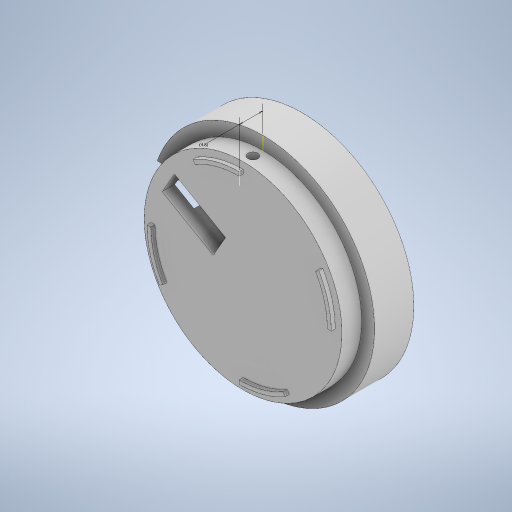
# Autodesk Inventor part: PiezoMount
Saved by Autodesk Inventor 2023 (Build 270158000, 158)
## iProperties
Created: 2023-02-27
Part Number: PiezoMount
Material: Generic
Document SubType Name: Modeling
Designer: maste
Density: 1 g/cm^3
Appearance: Default
Author: maste
Autodesk Inventor part; units mm, degrees
ref_plane "YZ Plane" through (0, 0, 0) normal (1, 0, 0) x (0, 1, 0)
ref_plane "XZ Plane" through (0, 0, 0) normal (0, 1, 0) x (-1, 0, 0)
ref_plane "XY Plane" through (0, 0, 0) normal (0, 0, 1) x (1, 0, 0)
sketch "Sketch1" plane through (0, 0, 0) normal (0, 0, 1) x (1, 0, 0)
  circle A0 centre (0, 0) radius 20.125
  dimension "d2" = 40.25
  constraints: 1 centre point, 1 coincident
  measures "d2" diameter of A0
extrude "piezo surface" add sketch "Sketch1" along normal blind 1
sketch "Sketch4" plane through (0, 0, 0) normal (0, 0, -1) x (-1, 0, 0)
  circle A0 centre (0, 0) radius 20.125 projected
extrude "Depth extension to surface" add sketch "Sketch4" along normal blind 6
sketch "Sketch2" plane through (0, 0, 1) normal (0, 0, 1) x (1, 0, 0)
  circle A0 centre (0, 0) radius 17.95
  circle A1 centre (0, 0) radius 18.75
  line L0 (0, 0) -> (18.75, 0)
  arc A2 (18.75, 0) -> (16.238, 9.375) centre (0, 0) ccw
  line L1 (0, 0) -> (16.238, 9.375) construction
  line L2 (0, 0) -> (18.75, 0) construction
  line L3 (16.238, 9.375) -> (15.5452, 8.975)
  line L4 (0, 0) -> (0, 18.75)
  line L5 (0, 0) -> (0, -18.75)
  line L6 (0, 0) -> (-18.75, 0)
  line L7 (0, 0) -> (-16.238, -9.375)
  line L8 (0, 0) -> (-9.375, 16.238)
  line L9 (0, 0) -> (9.375, -16.238)
  point P0 (17.95, 0)
  point P1 (8.975, -15.5452)
  point P2 (0, -17.95)
  point P3 (-15.5452, -8.975)
  point P4 (-17.95, 0)
  point P5 (-8.975, 15.5452)
  point P6 (0, 17.95)
  dimension "d3" = 35.9
  dimension "d4" = 37.5
  dimension "d5" = 30
  constraints: 20 end point, 4 point on line, 3 coincident, 2 perpendicular, 2 point on circle, 1 centre point, 1 horizontal, 1 vertical, 12 other
  measures "d5" angle of L2 L1
extrude "Diaphragm support" add sketch "Sketch2" along normal blind 0.8 contours A0 L3 A1 L0 | L9 A1 L5 A0 | A0 L8 A1 L4 | A0 L7 A1 L6
sketch "Sketch3" plane through (0, 0, 1) normal (0, 0, 1) x (1, 0, 0)
  line L0 (0, 0) -> (8.975, -15.5452)
  arc A0 (17.95, 0) -> (15.5452, 8.975) centre (0, 0) ccw projected
  line L1 (0, 0) -> (17.95, 0)
  arc A1 (0, -17.95) -> (8.975, -15.5452) centre (0, 0) ccw projected
  line L2 (8.975, -15.5452) -> (17.95, 0)
  line L3 (13.4625, -7.7726) -> (0, 0)
  line L4 (13.4625, -7.7726) -> (4.8022, -2.7726)
  line L5 (13.4625, -7.7726) -> (4.8022, -2.7726)
  line L6 (13.4625, -7.7726) -> (4.8022, -2.7726)
  line L7 (4.8022, -2.7726) -> (6.0522, -0.6075)
  line L8 (6.0522, -0.6075) -> (14.7125, -5.6075)
  line L9 (14.7125, -5.6075) -> (13.4625, -7.7726)
  line L10 (13.4625, -7.7726) -> (4.8022, -2.7726)
  line L11 (4.8022, -2.7726) -> (3.5522, -4.9376)
  line L12 (3.5522, -4.9376) -> (12.2125, -9.9376)
  line L13 (12.2125, -9.9376) -> (13.4625, -7.7726)
  line L14 (12.2125, -9.9376) -> (14.7125, -5.6075)
  line L15 (14.7125, -5.6075) -> (16.4446, -6.6075)
  line L16 (16.4446, -6.6075) -> (13.9446, -10.9376)
  line L17 (13.9446, -10.9376) -> (12.2125, -9.9376)
  line L18 (15.1946, -8.7726) -> (-15.1943, 8.7724)
  line L19 (-15.1943, 8.7724) -> (-4.802, 2.7724)
  line L20 (-4.802, 2.7724) -> (-3.552, 4.9375)
  line L21 (-3.552, 4.9375) -> (-13.9443, 10.9375)
  line L22 (-13.9443, 10.9375) -> (-15.1943, 8.7724)
  line L23 (-15.1943, 8.7724) -> (-4.802, 2.7724)
  line L24 (-4.802, 2.7724) -> (-6.052, 0.6074)
  line L25 (-6.052, 0.6074) -> (-16.4443, 6.6074)
  line L26 (-16.4443, 6.6074) -> (-15.1943, 8.7724)
  point P0 (14.7125, -5.6075)
  point P1 (12.2125, -9.9376)
  point P2 (12.2125, -9.9376)
  dimension "d37" = 10
  dimension "d38" = 2.5
  dimension "d39" = 2.5
  dimension "d40" = 2
  dimension "d49" = 10
  dimension "d50" = 35.09
  dimension "d51" = 12
  constraints: 54 end point, 10 parallel, 5 collinear, 5 perpendicular, 3 point on line, 2 midpoint
  measures "d37" distance of L3.start L4.end
  measures "d38" distance of L4.end L7.end
  measures "d39" distance of L11.end L4.end
  measures "d40" distance of L8.end L15.end
  measures "d49" distance between parallel lines of L11 L13
  measures "d50" distance of L18.start L18.end
  measures "d51" distance of L18.end L19.end
extrude "Microphone Wire Hole" cut sketch "Sketch3" against normal blind 14 contours L24 L25 L26 L18 | L18 L22 L21 L20
sketch "Sketch5" plane through (0, 0, -6) normal (0, 0, -1) x (-1, 0, 0)
  line L0 (12.5, -12.5) -> (-12.5, -12.5)
  line L1 (-12.5, -12.5) -> (-12.5, 12.5)
  line L2 (-12.5, 12.5) -> (12.5, 12.5)
  line L3 (12.5, 12.5) -> (12.5, -12.5)
  line L4 (12.5, -12.5) -> (-12.5, 12.5) construction
  line L5 (-12.5, -12.5) -> (12.5, 12.5) construction
  point P0 (0, 0)
  dimension "d18" = 25
  dimension "d19" = 25
  constraints: 12 end point, 2 midpoint, 2 parallel, 1 horizontal, 1 perpendicular
  measures "d18" distance of L0.start L0.end
  measures "d19" distance of L0.end L1.end
extrude "Circuit chamber" cut sketch "Sketch5" against normal blind 3
sketch "Sketch6" plane through (-12.5, -12.5, -6) normal (1, 0, 0) x (0, 0, -1)
  line L0 (0, 25) -> (0, 22.6036) projected
  line L1 (0, 25) -> (-3, 25) projected
  line L2 (-3, 25) -> (-3, 22.6036) projected
  line L3 (0, 0) -> (-3, 0) projected
  line L4 (-4.5, 5) -> (0, 5)
  line L5 (0, 5) -> (0, 20)
  line L6 (0, 20) -> (-4.5, 20)
  line L7 (-4.5, 20) -> (-4.5, 5)
  line L8 (-4.5, 5) -> (0, 20) construction
  line L9 (0, 5) -> (-4.5, 20) construction
  line L10 (0, 22.6036) -> (-3, 22.6036) projected
  line L11 (-3, 16.8301) -> (0, 16.8301) projected
  line L12 (-3, 16.8301) -> (-3, 0) projected
  line L13 (0, 16.8301) -> (0, 0) projected
  point P0 (-6, 12.5)
  point P1 (-2.25, 12.5)
  point P2 (-3, 20)
  point P3 (-3, 5)
  point P4 (0, 5)
  dimension "d22" = 15
  dimension "d45" = 5
  constraints: 12 end point, 2 midpoint, 2 parallel, 1 perpendicular
  measures "d22" distance of L5.end L4.end
  measures "d45" distance between parallel lines of L1 L6
extrude "port vent" cut sketch "Sketch6" against normal blind 30 contours L0 L10 L2 L1 | L4 L12 L11 L5 | L4 L7 L6 L5 L11 L12
sketch "Sketch7" plane through (0, 0, -6) normal (0, 0, -1) x (-1, 0, 0)
  line L0 (0, 0) -> (0, -17.5)
  line L1 (0, 0) -> (0, 17.5)
  dimension "d25" = 17.5
  dimension "d26" = 17.5
  constraints: 4 end point, 2 coincident, 2 vertical
  measures "d25" distance of L0.start L0.end
  measures "d26" distance of L0.start L1.end
hole "screw holes" at (0, 17.5, -6) at (0, -17.5, -6) direction (0, 0, 1) diameter 2.5 depth 4 tip angle 118
sketch "Sketch8" plane through (0, 0, -6) normal (0, 0, -1) x (-1, 0, 0)
  circle A0 centre (0, 0) radius 22.75
  line L0 (15.9289, 7.5) -> (18.6753, 7.5) projected
  line L1 (18.6753, 7.5) -> (21.4782, 7.5)
  arc A1 (18.6753, 7.5) -> (18.6753, -7.5) centre (0, 0) ccw projected
  line L2 (18.6753, -7.5) -> (21.4782, -7.5)
  point P0 (12.5, 7.5)
  dimension "d34" = 45.5
  constraints: 4 end point, 2 point on circle, 1 centre point, 1 coincident, 1 collinear, 1 parallel
  measures "d34" diameter of A0
extrude "Rim for flush with diaphragm lock" add sketch "Sketch8" against normal blind 3 contours L1 A1 L2 A0 picked at (-21.7141, -0.803)
sketch "Sketch9" plane through (0, 0, 0) normal (0, 1, 0) x (-1, 0, 0)
  line L0 (12.5, -3) -> (-12.5, -3) projected
  line L1 (0, -3) -> (0, -1)
  circle A0 centre (0, -1) radius 1
  point P0 (0, 0)
  dimension "d41" = 2
  dimension "d42" = 2
  constraints: 2 end point, 1 centre point, 1 coincident, 1 midpoint, 1 vertical
  measures "d41" distance of L1.start L1.end
  measures "d42" diameter of A0
extrude "Extrusion8" cut sketch "Sketch9" along normal mid plane 100
sketch "Sketch10" plane through (0, 0, -6) normal (0, 0, -1) x (-1, 0, 0)
  circle A0 centre (0, 17.5) radius 1.25 projected
  circle A1 centre (0, -17.5) radius 1.25 projected
  line L0 (15.9289, 7.5) -> (21.4782, 7.5) projected
  arc A2 (21.4782, 7.5) -> (21.4782, -7.5) centre (0, 0) ccw projected
  line L1 (21.4782, -7.5) -> (12.5, -7.5) projected
  line L2 (12.5, -7.5) -> (12.5, -12.5) projected
  line L3 (12.5, -12.5) -> (-12.5, -12.5) projected
  line L4 (-12.5, -12.5) -> (-12.5, 12.5) projected
  line L5 (-12.5, 12.5) -> (15.7723, 12.5) projected
  arc A3 (17.405, 10.1036) -> (15.7723, 12.5) centre (0, 0) ccw projected
  line L6 (17.405, 10.1036) -> (14.4257, 10.1036) projected
  line L7 (14.4257, 10.1036) -> (15.9289, 7.5) projected
extrude "Extrusion9" add sketch "Sketch10" along normal blind 5
sketch "Sketch11" plane through (0, 0, 0) normal (1, 0, 0) x (0, 1, 0)
  line L0 (18.75, 1.8) -> (16.238, 1.8) projected
  line L1 (22.75, -3) -> (-22.75, -3) projected
  point P0 (0, 0)
  point P1 (-7.5, -3)
  point P2 (7.5, -3)
  dimension "d52" = 4.8
  measures "d52" distance between parallel lines of L0 L1
body "Solid1"
